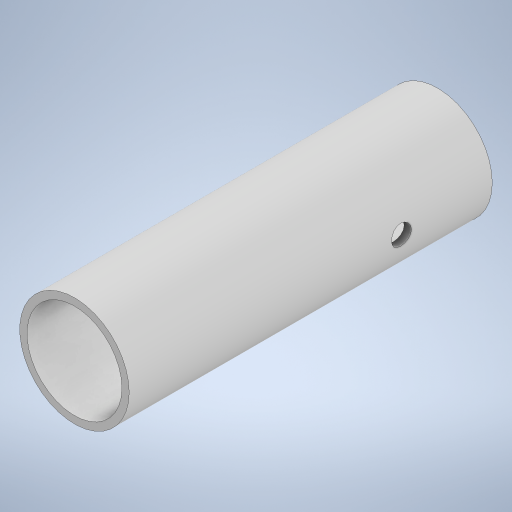
# Autodesk Inventor part: rura do spawania
Saved by Autodesk Inventor 2024 (Build 280153000, 153)
## iProperties
Created: 2024-12-02
Part Number: rura do spawania
Material: Generic
Document SubType Name: Modeling
Designer: Admin
Density: 1 g/cm^3
Appearance: Default
Author: Admin
Autodesk Inventor part; units mm, degrees
ref_plane "YZ Plane" through (0, 0, 0) normal (1, 0, 0) x (0, 1, 0)
ref_plane "XZ Plane" through (0, 0, 0) normal (0, 1, 0) x (-1, 0, 0)
ref_plane "XY Plane" through (0, 0, 0) normal (0, 0, 1) x (1, 0, 0)
sketch "Sketch1" plane through (0, 0, 0) normal (0, 0, 1) x (1, 0, 0)
  circle A0 centre (0, 0) radius 30.15
  dimension "d0" = 60.3
  constraints: 1 centre point, 1 coincident
  measures "d0" diameter of A0
extrude "Extrusion1" add sketch "Sketch1" along normal blind 200
sketch "Sketch2" plane through (0, 0, 200) normal (0, 0, 1) x (1, 0, 0)
  circle A0 centre (0, 0) radius 26.15
  dimension "d3" = 52.3
  constraints: 1 centre point, 1 coincident
  measures "d3" diameter of A0
extrude "Extrusion2" cut sketch "Sketch2" against normal blind 200
sketch "Sketch3" plane through (0, 0, 0) normal (1, 0, 0) x (0, 1, 0)
  circle A0 centre (0, 50) radius 5.5
  line L0 (30.15, 0) -> (-30.15, 0) projected
  point P0 (0, 0)
  dimension "d6" = 11
  dimension "d7" = 50
  constraints: 1 centre point
  measures "d6" diameter of A0
  measures "d7" distance from line of L0 A0.centre
extrude "Extrusion3" cut sketch "Sketch3" along normal through all both and the other way through all
body "Solid1"
